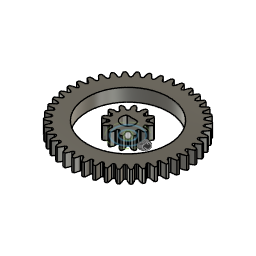
MVP miniaturisé (Autodesk Fusion 360 archive; units mm, degrees)
design "Roue dentée miniature"
description: Spur Gear; Module: 1.0; Num Teeth: 12; Pressure Angle: 20.0; Backlash: 0.00 mm
description: Spur Gear; Module: 1.0; Num Teeth: 42; Pressure Angle: 20.0; Backlash: 0.00 mm
Autodesk Fusion 360 part; units mm, degrees
(part 1 of 2)
sketch "Esquisse1" plane through (0, 0, 0) normal (0, 0, 1) x (1, 0, 0) in component "Spur Gear (12 teeth)"
  circle A0 centre (0, 0) radius 4.7492
  circle A1 centre (0, 0) radius 2.5
extrude "Extrusion1" add sketch "Esquisse1" along normal blind 4.7 makes body 1 in component "Spur Gear (12 teeth)"
sketch "Esquisse2" plane through (0, 0, 0) normal (0, 0, 1) x (1, 0, 0) in component "Spur Gear (12 teeth)"
  spline S0 degree 5 poles (5.5783, -0.8192) (5.5823, -0.8197) (5.5902, -0.8208) (5.6021, -0.8219) (5.6181, -0.8228) (5.6381, -0.8229) (5.6583, -0.8223) (5.6784, -0.8212) (5.6986, -0.8199) (5.7188, -0.8184) (5.7391, -0.8168) (5.7593, -0.8149) (5.7796, -0.8127) (5.7999, -0.8102) (5.8203, -0.8073) (5.8406, -0.8041) (5.861, -0.8006) (5.8814, -0.7969) (5.9018, -0.793) (5.9222, -0.7888) (5.9426, -0.7845) (5.9631, -0.7799) (5.9835, -0.7752) (6.0039, -0.7702) (6.0244, -0.765) (6.0448, -0.7596) (6.0653, -0.7539) (6.0857, -0.7481) (6.1061, -0.7421) (6.1266, -0.7359) (6.147, -0.7295) (6.1675, -0.7229) (6.1879, -0.7161) (6.2083, -0.7092) (6.2288, -0.7021) (6.2492, -0.6947) (6.2696, -0.6873) (6.29, -0.6796) (6.3104, -0.6717) (6.3308, -0.6637) (6.3512, -0.6555) (6.3715, -0.6472) (6.3919, -0.6387) (6.4122, -0.63) (6.4325, -0.6211) (6.4528, -0.6121) (6.4731, -0.6029) (6.4934, -0.5936) (6.5137, -0.5841) (6.5339, -0.5744) (6.5541, -0.5646) (6.5743, -0.5546) (6.5945, -0.5445) (6.6147, -0.5342) (6.6348, -0.5238) (6.655, -0.5132) (6.6751, -0.5024) (6.6951, -0.4915) (6.7152, -0.4805) (6.7352, -0.4693) (6.7552, -0.4579) (6.7752, -0.4464) (6.7952, -0.4348) (6.8151, -0.423) (6.835, -0.4111) (6.8549, -0.399) (6.8747, -0.3867) (6.8945, -0.3744) (6.9143, -0.3619) (6.9341, -0.3492) (6.9538, -0.3364) (6.9695, -0.3261) (6.9813, -0.3182) (6.9892, -0.313) (6.9931, -0.3103) knots 0 0 0 0 0 0 0.01428571 0.02857143 0.04285714 0.05714286 0.07142857 0.08571429 0.1 0.11428571 0.12857143 0.14285714 0.15714286 0.17142857 0.18571429 0.2 0.21428571 0.22857143 0.24285714 0.25714286 0.27142857 0.28571429 0.3 0.31428571 0.32857143 0.34285714 0.35714286 0.37142857 0.38571429 0.4 0.41428571 0.42857143 0.44285714 0.45714286 0.47142857 0.48571429 0.5 0.51428571 0.52857143 0.54285714 0.55714286 0.57142857 0.58571429 0.6 0.61428571 0.62857143 0.64285714 0.65714286 0.67142857 0.68571429 0.7 0.71428571 0.72857143 0.74285714 0.75714286 0.77142857 0.78571429 0.8 0.81428571 0.82857143 0.84285714 0.85714286 0.87142857 0.88571429 0.9 0.91428571 0.92857143 0.94285714 0.95714286 0.97142857 0.98571429 1 1 1 1 1 1
  spline S1 degree 5 poles (5.5783, 0.8192) (5.5823, 0.8197) (5.5902, 0.8208) (5.6021, 0.8219) (5.6181, 0.8228) (5.6381, 0.8229) (5.6583, 0.8223) (5.6784, 0.8212) (5.6986, 0.8199) (5.7188, 0.8184) (5.7391, 0.8168) (5.7593, 0.8149) (5.7796, 0.8127) (5.7999, 0.8102) (5.8203, 0.8073) (5.8406, 0.8041) (5.861, 0.8006) (5.8814, 0.7969) (5.9018, 0.793) (5.9222, 0.7888) (5.9426, 0.7845) (5.9631, 0.7799) (5.9835, 0.7752) (6.0039, 0.7702) (6.0244, 0.765) (6.0448, 0.7596) (6.0653, 0.7539) (6.0857, 0.7481) (6.1061, 0.7421) (6.1266, 0.7359) (6.147, 0.7295) (6.1675, 0.7229) (6.1879, 0.7161) (6.2083, 0.7092) (6.2288, 0.7021) (6.2492, 0.6947) (6.2696, 0.6873) (6.29, 0.6796) (6.3104, 0.6717) (6.3308, 0.6637) (6.3512, 0.6555) (6.3715, 0.6472) (6.3919, 0.6387) (6.4122, 0.63) (6.4325, 0.6211) (6.4528, 0.6121) (6.4731, 0.6029) (6.4934, 0.5936) (6.5137, 0.5841) (6.5339, 0.5744) (6.5541, 0.5646) (6.5743, 0.5546) (6.5945, 0.5445) (6.6147, 0.5342) (6.6348, 0.5238) (6.655, 0.5132) (6.6751, 0.5024) (6.6951, 0.4915) (6.7152, 0.4805) (6.7352, 0.4693) (6.7552, 0.4579) (6.7752, 0.4464) (6.7952, 0.4348) (6.8151, 0.423) (6.835, 0.4111) (6.8549, 0.399) (6.8747, 0.3867) (6.8945, 0.3744) (6.9143, 0.3619) (6.9341, 0.3492) (6.9538, 0.3364) (6.9695, 0.3261) (6.9813, 0.3182) (6.9892, 0.313) (6.9931, 0.3103) knots 0 0 0 0 0 0 0.01428571 0.02857143 0.04285714 0.05714286 0.07142857 0.08571429 0.1 0.11428571 0.12857143 0.14285714 0.15714286 0.17142857 0.18571429 0.2 0.21428571 0.22857143 0.24285714 0.25714286 0.27142857 0.28571429 0.3 0.31428571 0.32857143 0.34285714 0.35714286 0.37142857 0.38571429 0.4 0.41428571 0.42857143 0.44285714 0.45714286 0.47142857 0.48571429 0.5 0.51428571 0.52857143 0.54285714 0.55714286 0.57142857 0.58571429 0.6 0.61428571 0.62857143 0.64285714 0.65714286 0.67142857 0.68571429 0.7 0.71428571 0.72857143 0.74285714 0.75714286 0.77142857 0.78571429 0.8 0.81428571 0.82857143 0.84285714 0.85714286 0.87142857 0.88571429 0.9 0.91428571 0.92857143 0.94285714 0.95714286 0.97142857 0.98571429 1 1 1 1 1 1
  arc A0 (6.9931, -0.3103) -> (6.9931, 0.3103) centre (0, 0) ccw
  line L0 (4.6889, -0.69) -> (5.5783, -0.8192)
  line L1 (4.6889, 0.69) -> (5.5783, 0.8192)
  line L2 (4.6889, -0.69) -> (4.6889, 0.69)
  point P0 (5.6763, -0.8213)
  point P1 (5.7758, -0.8131)
  point P2 (5.8761, -0.7978)
  point P3 (5.977, -0.7767)
  point P4 (6.0784, -0.7502)
  point P5 (6.1802, -0.7187)
  point P6 (6.2821, -0.6825)
  point P7 (6.3842, -0.6419)
  point P8 (6.4862, -0.5969)
  point P9 (6.5882, -0.5477)
  point P10 (6.6899, -0.4943)
  point P11 (6.7914, -0.437)
  point P12 (6.8925, -0.3756)
  point P13 (5.6763, 0.8213)
  point P14 (5.7758, 0.8131)
  point P15 (5.8761, 0.7978)
  point P16 (5.977, 0.7767)
  point P17 (6.0784, 0.7502)
  point P18 (6.1802, 0.7187)
  point P19 (6.2821, 0.6825)
  point P20 (6.3842, 0.6419)
  point P21 (6.4862, 0.5969)
  point P22 (6.5882, 0.5477)
  point P23 (6.6899, 0.4943)
  point P24 (6.7914, 0.437)
  point P25 (6.8925, 0.3756)
extrude "Extrusion2" add sketch "Esquisse2" along normal blind 4.7 bodies 1 in component "Spur Gear (12 teeth)"
fillet "Congé1" radius 0.5 2 edges at (4.6986, -0.6914, 2.35) (4.6986, 0.6914, 2.35) on bodies 1 in component "Spur Gear (12 teeth)"
pattern_circular "Réseau C1" count 12 over 360 about axis through (0, 0, 0) along (0, 0, 1) of "Extrusion2", "Congé1" in component "Spur Gear (12 teeth)"
sketch "Esquisse3" plane through (0, 0, 0) normal (0, 0, 1) x (1, 0, 0) in component "Spur Gear (12 teeth)"
  circle A0 centre (0, 0) radius 6 construction
sketch "Esquisse2 (2)" plane through (0, 0, 0) normal (0, 0, -1) x (1, 0, 0)
  circle A0 centre (0, 0) radius 2.5
  arc A1 (3.2424, 4.0966) -> (3.2887, 3.4262) centre (3.635, 3.7869) ccw
  line L0 (3.2424, 4.0966) -> (3.4986, 4.4214)
  spline S0 degree 5 poles (3.4986, 4.4214) (3.5011, 4.4245) (3.5059, 4.4309) (3.5129, 4.4406) (3.5216, 4.454) (3.5317, 4.4713) (3.5412, 4.4891) (3.5504, 4.5071) (3.5594, 4.5252) (3.5682, 4.5434) (3.5769, 4.5618) (3.5854, 4.5803) (3.5936, 4.599) (3.6016, 4.6178) (3.6093, 4.6369) (3.6167, 4.6561) (3.6239, 4.6755) (3.6308, 4.695) (3.6376, 4.7146) (3.6442, 4.7344) (3.6507, 4.7542) (3.657, 4.7742) (3.6631, 4.7943) (3.669, 4.8144) (3.6747, 4.8348) (3.6802, 4.8552) (3.6856, 4.8757) (3.6907, 4.8963) (3.6957, 4.917) (3.7006, 4.9378) (3.7053, 4.9587) (3.7098, 4.9797) (3.7142, 5.0008) (3.7184, 5.022) (3.7224, 5.0432) (3.7263, 5.0646) (3.73, 5.086) (3.7335, 5.1075) (3.7369, 5.1291) (3.7402, 5.1508) (3.7433, 5.1725) (3.7462, 5.1943) (3.749, 5.2162) (3.7517, 5.2381) (3.7542, 5.2602) (3.7565, 5.2823) (3.7587, 5.3044) (3.7608, 5.3267) (3.7627, 5.349) (3.7644, 5.3713) (3.766, 5.3937) (3.7675, 5.4162) (3.7688, 5.4388) (3.77, 5.4614) (3.771, 5.4841) (3.7719, 5.5068) (3.7726, 5.5296) (3.7732, 5.5524) (3.7737, 5.5753) (3.774, 5.5982) (3.7742, 5.6212) (3.7742, 5.6443) (3.7741, 5.6674) (3.7739, 5.6906) (3.7735, 5.7138) (3.773, 5.737) (3.7723, 5.7603) (3.7715, 5.7836) (3.7705, 5.807) (3.7694, 5.8305) (3.7682, 5.8539) (3.7671, 5.8728) (3.7663, 5.8869) (3.7656, 5.8963) (3.7653, 5.901) knots 0 0 0 0 0 0 0.01428571 0.02857143 0.04285714 0.05714286 0.07142857 0.08571429 0.1 0.11428571 0.12857143 0.14285714 0.15714286 0.17142857 0.18571429 0.2 0.21428571 0.22857143 0.24285714 0.25714286 0.27142857 0.28571429 0.3 0.31428571 0.32857143 0.34285714 0.35714286 0.37142857 0.38571429 0.4 0.41428571 0.42857143 0.44285714 0.45714286 0.47142857 0.48571429 0.5 0.51428571 0.52857143 0.54285714 0.55714286 0.57142857 0.58571429 0.6 0.61428571 0.62857143 0.64285714 0.65714286 0.67142857 0.68571429 0.7 0.71428571 0.72857143 0.74285714 0.75714286 0.77142857 0.78571429 0.8 0.81428571 0.82857143 0.84285714 0.85714286 0.87142857 0.88571429 0.9 0.91428571 0.92857143 0.94285714 0.95714286 0.97142857 0.98571429 1 1 1 1 1 1
  arc A2 (3.7653, 5.901) -> (3.2278, 6.2114) centre (0, 0) ccw
  spline S1 degree 5 poles (2.0798, 5.2406) (2.0812, 5.2443) (2.0843, 5.2517) (2.0893, 5.2626) (2.0965, 5.2768) (2.1064, 5.2942) (2.117, 5.3113) (2.128, 5.3283) (2.1393, 5.3451) (2.1506, 5.3619) (2.1622, 5.3786) (2.174, 5.3952) (2.186, 5.4117) (2.1983, 5.428) (2.211, 5.4442) (2.2239, 5.4602) (2.2372, 5.4761) (2.2506, 5.4919) (2.2642, 5.5076) (2.278, 5.5232) (2.2919, 5.5387) (2.3061, 5.5541) (2.3204, 5.5694) (2.3349, 5.5846) (2.3497, 5.5997) (2.3646, 5.6147) (2.3797, 5.6296) (2.395, 5.6444) (2.4104, 5.6591) (2.426, 5.6737) (2.4418, 5.6882) (2.4577, 5.7026) (2.4738, 5.717) (2.49, 5.7312) (2.5064, 5.7453) (2.5229, 5.7593) (2.5396, 5.7733) (2.5565, 5.7871) (2.5735, 5.8008) (2.5906, 5.8145) (2.6079, 5.828) (2.6253, 5.8415) (2.6428, 5.8549) (2.6605, 5.8681) (2.6784, 5.8813) (2.6963, 5.8944) (2.7144, 5.9074) (2.7326, 5.9203) (2.751, 5.9331) (2.7695, 5.9458) (2.7881, 5.9584) (2.8068, 5.9709) (2.8257, 5.9833) (2.8447, 5.9956) (2.8638, 6.0078) (2.8831, 6.02) (2.9024, 6.032) (2.9219, 6.0439) (2.9415, 6.0558) (2.9612, 6.0675) (2.981, 6.0792) (3.001, 6.0907) (3.0211, 6.1022) (3.0412, 6.1135) (3.0615, 6.1248) (3.0819, 6.136) (3.1024, 6.147) (3.123, 6.158) (3.1438, 6.1689) (3.1646, 6.1797) (3.1856, 6.1903) (3.2024, 6.1988) (3.2151, 6.2051) (3.2235, 6.2093) (3.2278, 6.2114) knots 0 0 0 0 0 0 0.01428571 0.02857143 0.04285714 0.05714286 0.07142857 0.08571429 0.1 0.11428571 0.12857143 0.14285714 0.15714286 0.17142857 0.18571429 0.2 0.21428571 0.22857143 0.24285714 0.25714286 0.27142857 0.28571429 0.3 0.31428571 0.32857143 0.34285714 0.35714286 0.37142857 0.38571429 0.4 0.41428571 0.42857143 0.44285714 0.45714286 0.47142857 0.48571429 0.5 0.51428571 0.52857143 0.54285714 0.55714286 0.57142857 0.58571429 0.6 0.61428571 0.62857143 0.64285714 0.65714286 0.67142857 0.68571429 0.7 0.71428571 0.72857143 0.74285714 0.75714286 0.77142857 0.78571429 0.8 0.81428571 0.82857143 0.84285714 0.85714286 0.87142857 0.88571429 0.9 0.91428571 0.92857143 0.94285714 0.95714286 0.97142857 0.98571429 1 1 1 1 1 1
  line L1 (2.0798, 5.2406) -> (1.9265, 4.8563)
  arc A3 (1.3228, 4.5613) -> (1.9265, 4.8563) centre (1.4621, 5.0415) ccw
  arc A4 (1.3228, 4.5613) -> (1.135, 4.6116) centre (0, 0) ccw
  arc A5 (0.7597, 5.1689) -> (1.135, 4.6116) centre (1.2545, 5.0971) ccw
  line L2 (0.7597, 5.1689) -> (0.8192, 5.5783)
  spline S2 degree 5 poles (0.8192, 5.5783) (0.8197, 5.5823) (0.8208, 5.5902) (0.8219, 5.6021) (0.8228, 5.6181) (0.8229, 5.6381) (0.8223, 5.6583) (0.8212, 5.6784) (0.8199, 5.6986) (0.8184, 5.7188) (0.8168, 5.7391) (0.8149, 5.7593) (0.8127, 5.7796) (0.8102, 5.7999) (0.8073, 5.8203) (0.8041, 5.8406) (0.8006, 5.861) (0.7969, 5.8814) (0.793, 5.9018) (0.7888, 5.9222) (0.7845, 5.9426) (0.7799, 5.9631) (0.7752, 5.9835) (0.7702, 6.0039) (0.765, 6.0244) (0.7596, 6.0448) (0.7539, 6.0653) (0.7481, 6.0857) (0.7421, 6.1061) (0.7359, 6.1266) (0.7295, 6.147) (0.7229, 6.1675) (0.7161, 6.1879) (0.7092, 6.2083) (0.7021, 6.2288) (0.6947, 6.2492) (0.6873, 6.2696) (0.6796, 6.29) (0.6717, 6.3104) (0.6637, 6.3308) (0.6555, 6.3512) (0.6472, 6.3715) (0.6387, 6.3919) (0.63, 6.4122) (0.6211, 6.4325) (0.6121, 6.4528) (0.6029, 6.4731) (0.5936, 6.4934) (0.5841, 6.5137) (0.5744, 6.5339) (0.5646, 6.5541) (0.5546, 6.5743) (0.5445, 6.5945) (0.5342, 6.6147) (0.5238, 6.6348) (0.5132, 6.655) (0.5024, 6.6751) (0.4915, 6.6951) (0.4805, 6.7152) (0.4693, 6.7352) (0.4579, 6.7552) (0.4464, 6.7752) (0.4348, 6.7952) (0.423, 6.8151) (0.4111, 6.835) (0.399, 6.8549) (0.3867, 6.8747) (0.3744, 6.8945) (0.3619, 6.9143) (0.3492, 6.9341) (0.3364, 6.9538) (0.3261, 6.9695) (0.3182, 6.9813) (0.313, 6.9892) (0.3103, 6.9931) knots 0 0 0 0 0 0 0.01428571 0.02857143 0.04285714 0.05714286 0.07142857 0.08571429 0.1 0.11428571 0.12857143 0.14285714 0.15714286 0.17142857 0.18571429 0.2 0.21428571 0.22857143 0.24285714 0.25714286 0.27142857 0.28571429 0.3 0.31428571 0.32857143 0.34285714 0.35714286 0.37142857 0.38571429 0.4 0.41428571 0.42857143 0.44285714 0.45714286 0.47142857 0.48571429 0.5 0.51428571 0.52857143 0.54285714 0.55714286 0.57142857 0.58571429 0.6 0.61428571 0.62857143 0.64285714 0.65714286 0.67142857 0.68571429 0.7 0.71428571 0.72857143 0.74285714 0.75714286 0.77142857 0.78571429 0.8 0.81428571 0.82857143 0.84285714 0.85714286 0.87142857 0.88571429 0.9 0.91428571 0.92857143 0.94285714 0.95714286 0.97142857 0.98571429 1 1 1 1 1 1
  arc A6 (0.3103, 6.9931) -> (-0.3103, 6.9931) centre (0, 0) ccw
  spline S3 degree 5 poles (-0.8192, 5.5783) (-0.8197, 5.5823) (-0.8208, 5.5902) (-0.8219, 5.6021) (-0.8228, 5.6181) (-0.8229, 5.6381) (-0.8223, 5.6583) (-0.8212, 5.6784) (-0.8199, 5.6986) (-0.8184, 5.7188) (-0.8168, 5.7391) (-0.8149, 5.7593) (-0.8127, 5.7796) (-0.8102, 5.7999) (-0.8073, 5.8203) (-0.8041, 5.8406) (-0.8006, 5.861) (-0.7969, 5.8814) (-0.793, 5.9018) (-0.7888, 5.9222) (-0.7845, 5.9426) (-0.7799, 5.9631) (-0.7752, 5.9835) (-0.7702, 6.0039) (-0.765, 6.0244) (-0.7596, 6.0448) (-0.7539, 6.0653) (-0.7481, 6.0857) (-0.7421, 6.1061) (-0.7359, 6.1266) (-0.7295, 6.147) (-0.7229, 6.1675) (-0.7161, 6.1879) (-0.7092, 6.2083) (-0.7021, 6.2288) (-0.6947, 6.2492) (-0.6873, 6.2696) (-0.6796, 6.29) (-0.6717, 6.3104) (-0.6637, 6.3308) (-0.6555, 6.3512) (-0.6472, 6.3715) (-0.6387, 6.3919) (-0.63, 6.4122) (-0.6211, 6.4325) (-0.6121, 6.4528) (-0.6029, 6.4731) (-0.5936, 6.4934) (-0.5841, 6.5137) (-0.5744, 6.5339) (-0.5646, 6.5541) (-0.5546, 6.5743) (-0.5445, 6.5945) (-0.5342, 6.6147) (-0.5238, 6.6348) (-0.5132, 6.655) (-0.5024, 6.6751) (-0.4915, 6.6951) (-0.4805, 6.7152) (-0.4693, 6.7352) (-0.4579, 6.7552) (-0.4464, 6.7752) (-0.4348, 6.7952) (-0.423, 6.8151) (-0.4111, 6.835) (-0.399, 6.8549) (-0.3867, 6.8747) (-0.3744, 6.8945) (-0.3619, 6.9143) (-0.3492, 6.9341) (-0.3364, 6.9538) (-0.3261, 6.9695) (-0.3182, 6.9813) (-0.313, 6.9892) (-0.3103, 6.9931) knots 0 0 0 0 0 0 0.01428571 0.02857143 0.04285714 0.05714286 0.07142857 0.08571429 0.1 0.11428571 0.12857143 0.14285714 0.15714286 0.17142857 0.18571429 0.2 0.21428571 0.22857143 0.24285714 0.25714286 0.27142857 0.28571429 0.3 0.31428571 0.32857143 0.34285714 0.35714286 0.37142857 0.38571429 0.4 0.41428571 0.42857143 0.44285714 0.45714286 0.47142857 0.48571429 0.5 0.51428571 0.52857143 0.54285714 0.55714286 0.57142857 0.58571429 0.6 0.61428571 0.62857143 0.64285714 0.65714286 0.67142857 0.68571429 0.7 0.71428571 0.72857143 0.74285714 0.75714286 0.77142857 0.78571429 0.8 0.81428571 0.82857143 0.84285714 0.85714286 0.87142857 0.88571429 0.9 0.91428571 0.92857143 0.94285714 0.95714286 0.97142857 0.98571429 1 1 1 1 1 1
  line L3 (-0.8192, 5.5783) -> (-0.7597, 5.1689)
  arc A7 (-1.135, 4.6116) -> (-0.7597, 5.1689) centre (-1.2545, 5.0971) ccw
  arc A8 (-1.135, 4.6116) -> (-1.3228, 4.5613) centre (0, 0) ccw
  arc A9 (-1.9265, 4.8563) -> (-1.3228, 4.5613) centre (-1.4621, 5.0415) ccw
  line L4 (-1.9265, 4.8563) -> (-2.0798, 5.2406)
  spline S4 degree 5 poles (-2.0798, 5.2406) (-2.0812, 5.2443) (-2.0843, 5.2517) (-2.0893, 5.2626) (-2.0965, 5.2768) (-2.1064, 5.2942) (-2.117, 5.3113) (-2.128, 5.3283) (-2.1393, 5.3451) (-2.1506, 5.3619) (-2.1622, 5.3786) (-2.174, 5.3952) (-2.186, 5.4117) (-2.1983, 5.428) (-2.211, 5.4442) (-2.2239, 5.4602) (-2.2372, 5.4761) (-2.2506, 5.4919) (-2.2642, 5.5076) (-2.278, 5.5232) (-2.2919, 5.5387) (-2.3061, 5.5541) (-2.3204, 5.5694) (-2.3349, 5.5846) (-2.3497, 5.5997) (-2.3646, 5.6147) (-2.3797, 5.6296) (-2.395, 5.6444) (-2.4104, 5.6591) (-2.426, 5.6737) (-2.4418, 5.6882) (-2.4577, 5.7026) (-2.4738, 5.717) (-2.49, 5.7312) (-2.5064, 5.7453) (-2.5229, 5.7593) (-2.5396, 5.7733) (-2.5565, 5.7871) (-2.5735, 5.8008) (-2.5906, 5.8145) (-2.6079, 5.828) (-2.6253, 5.8415) (-2.6428, 5.8549) (-2.6605, 5.8681) (-2.6784, 5.8813) (-2.6963, 5.8944) (-2.7144, 5.9074) (-2.7326, 5.9203) (-2.751, 5.9331) (-2.7695, 5.9458) (-2.7881, 5.9584) (-2.8068, 5.9709) (-2.8257, 5.9833) (-2.8447, 5.9956) (-2.8638, 6.0078) (-2.8831, 6.02) (-2.9024, 6.032) (-2.9219, 6.0439) (-2.9415, 6.0558) (-2.9612, 6.0675) (-2.981, 6.0792) (-3.001, 6.0907) (-3.0211, 6.1022) (-3.0412, 6.1135) (-3.0615, 6.1248) (-3.0819, 6.136) (-3.1024, 6.147) (-3.123, 6.158) (-3.1438, 6.1689) (-3.1646, 6.1797) (-3.1856, 6.1903) (-3.2024, 6.1988) (-3.2151, 6.2051) (-3.2235, 6.2093) (-3.2278, 6.2114) knots 0 0 0 0 0 0 0.01428571 0.02857143 0.04285714 0.05714286 0.07142857 0.08571429 0.1 0.11428571 0.12857143 0.14285714 0.15714286 0.17142857 0.18571429 0.2 0.21428571 0.22857143 0.24285714 0.25714286 0.27142857 0.28571429 0.3 0.31428571 0.32857143 0.34285714 0.35714286 0.37142857 0.38571429 0.4 0.41428571 0.42857143 0.44285714 0.45714286 0.47142857 0.48571429 0.5 0.51428571 0.52857143 0.54285714 0.55714286 0.57142857 0.58571429 0.6 0.61428571 0.62857143 0.64285714 0.65714286 0.67142857 0.68571429 0.7 0.71428571 0.72857143 0.74285714 0.75714286 0.77142857 0.78571429 0.8 0.81428571 0.82857143 0.84285714 0.85714286 0.87142857 0.88571429 0.9 0.91428571 0.92857143 0.94285714 0.95714286 0.97142857 0.98571429 1 1 1 1 1 1
  arc A10 (-3.2278, 6.2114) -> (-3.7653, 5.901) centre (0, 0) ccw
  spline S5 degree 5 poles (-3.4986, 4.4214) (-3.5011, 4.4245) (-3.5059, 4.4309) (-3.5129, 4.4406) (-3.5216, 4.454) (-3.5317, 4.4713) (-3.5412, 4.4891) (-3.5504, 4.5071) (-3.5594, 4.5252) (-3.5682, 4.5434) (-3.5769, 4.5618) (-3.5854, 4.5803) (-3.5936, 4.599) (-3.6016, 4.6178) (-3.6093, 4.6369) (-3.6167, 4.6561) (-3.6239, 4.6755) (-3.6308, 4.695) (-3.6376, 4.7146) (-3.6442, 4.7344) (-3.6507, 4.7542) (-3.657, 4.7742) (-3.6631, 4.7943) (-3.669, 4.8144) (-3.6747, 4.8348) (-3.6802, 4.8552) (-3.6856, 4.8757) (-3.6907, 4.8963) (-3.6957, 4.917) (-3.7006, 4.9378) (-3.7053, 4.9587) (-3.7098, 4.9797) (-3.7142, 5.0008) (-3.7184, 5.022) (-3.7224, 5.0432) (-3.7263, 5.0646) (-3.73, 5.086) (-3.7335, 5.1075) (-3.7369, 5.1291) (-3.7402, 5.1508) (-3.7433, 5.1725) (-3.7462, 5.1943) (-3.749, 5.2162) (-3.7517, 5.2381) (-3.7542, 5.2602) (-3.7565, 5.2823) (-3.7587, 5.3044) (-3.7608, 5.3267) (-3.7627, 5.349) (-3.7644, 5.3713) (-3.766, 5.3937) (-3.7675, 5.4162) (-3.7688, 5.4388) (-3.77, 5.4614) (-3.771, 5.4841) (-3.7719, 5.5068) (-3.7726, 5.5296) (-3.7732, 5.5524) (-3.7737, 5.5753) (-3.774, 5.5982) (-3.7742, 5.6212) (-3.7742, 5.6443) (-3.7741, 5.6674) (-3.7739, 5.6906) (-3.7735, 5.7138) (-3.773, 5.737) (-3.7723, 5.7603) (-3.7715, 5.7836) (-3.7705, 5.807) (-3.7694, 5.8305) (-3.7682, 5.8539) (-3.7671, 5.8728) (-3.7663, 5.8869) (-3.7656, 5.8963) (-3.7653, 5.901) knots 0 0 0 0 0 0 0.01428571 0.02857143 0.04285714 0.05714286 0.07142857 0.08571429 0.1 0.11428571 0.12857143 0.14285714 0.15714286 0.17142857 0.18571429 0.2 0.21428571 0.22857143 0.24285714 0.25714286 0.27142857 0.28571429 0.3 0.31428571 0.32857143 0.34285714 0.35714286 0.37142857 0.38571429 0.4 0.41428571 0.42857143 0.44285714 0.45714286 0.47142857 0.48571429 0.5 0.51428571 0.52857143 0.54285714 0.55714286 0.57142857 0.58571429 0.6 0.61428571 0.62857143 0.64285714 0.65714286 0.67142857 0.68571429 0.7 0.71428571 0.72857143 0.74285714 0.75714286 0.77142857 0.78571429 0.8 0.81428571 0.82857143 0.84285714 0.85714286 0.87142857 0.88571429 0.9 0.91428571 0.92857143 0.94285714 0.95714286 0.97142857 0.98571429 1 1 1 1 1 1
  line L5 (-3.4986, 4.4214) -> (-3.2424, 4.0966)
  arc A11 (-3.2887, 3.4262) -> (-3.2424, 4.0966) centre (-3.635, 3.7869) ccw
  arc A12 (-3.2887, 3.4262) -> (-3.4262, 3.2887) centre (0, 0) ccw
  arc A13 (-4.0966, 3.2424) -> (-3.4262, 3.2887) centre (-3.7869, 3.635) ccw
  line L6 (-4.0966, 3.2424) -> (-4.4214, 3.4986)
  spline S6 degree 5 poles (-4.4214, 3.4986) (-4.4245, 3.5011) (-4.4309, 3.5059) (-4.4406, 3.5129) (-4.454, 3.5216) (-4.4713, 3.5317) (-4.4891, 3.5412) (-4.5071, 3.5504) (-4.5252, 3.5594) (-4.5434, 3.5682) (-4.5618, 3.5769) (-4.5803, 3.5854) (-4.599, 3.5936) (-4.6178, 3.6016) (-4.6369, 3.6093) (-4.6561, 3.6167) (-4.6755, 3.6239) (-4.695, 3.6308) (-4.7146, 3.6376) (-4.7344, 3.6442) (-4.7542, 3.6507) (-4.7742, 3.657) (-4.7943, 3.6631) (-4.8144, 3.669) (-4.8348, 3.6747) (-4.8552, 3.6802) (-4.8757, 3.6856) (-4.8963, 3.6907) (-4.917, 3.6957) (-4.9378, 3.7006) (-4.9587, 3.7053) (-4.9797, 3.7098) (-5.0008, 3.7142) (-5.022, 3.7184) (-5.0432, 3.7224) (-5.0646, 3.7263) (-5.086, 3.73) (-5.1075, 3.7335) (-5.1291, 3.7369) (-5.1508, 3.7402) (-5.1725, 3.7433) (-5.1943, 3.7462) (-5.2162, 3.749) (-5.2381, 3.7517) (-5.2602, 3.7542) (-5.2823, 3.7565) (-5.3044, 3.7587) (-5.3267, 3.7608) (-5.349, 3.7627) (-5.3713, 3.7644) (-5.3937, 3.766) (-5.4162, 3.7675) (-5.4388, 3.7688) (-5.4614, 3.77) (-5.4841, 3.771) (-5.5068, 3.7719) (-5.5296, 3.7726) (-5.5524, 3.7732) (-5.5753, 3.7737) (-5.5982, 3.774) (-5.6212, 3.7742) (-5.6443, 3.7742) (-5.6674, 3.7741) (-5.6906, 3.7739) (-5.7138, 3.7735) (-5.737, 3.773) (-5.7603, 3.7723) (-5.7836, 3.7715) (-5.807, 3.7705) (-5.8305, 3.7694) (-5.8539, 3.7682) (-5.8728, 3.7671) (-5.8869, 3.7663) (-5.8963, 3.7656) (-5.901, 3.7653) knots 0 0 0 0 0 0 0.01428571 0.02857143 0.04285714 0.05714286 0.07142857 0.08571429 0.1 0.11428571 0.12857143 0.14285714 0.15714286 0.17142857 0.18571429 0.2 0.21428571 0.22857143 0.24285714 0.25714286 0.27142857 0.28571429 0.3 0.31428571 0.32857143 0.34285714 0.35714286 0.37142857 0.38571429 0.4 0.41428571 0.42857143 0.44285714 0.45714286 0.47142857 0.48571429 0.5 0.51428571 0.52857143 0.54285714 0.55714286 0.57142857 0.58571429 0.6 0.61428571 0.62857143 0.64285714 0.65714286 0.67142857 0.68571429 0.7 0.71428571 0.72857143 0.74285714 0.75714286 0.77142857 0.78571429 0.8 0.81428571 0.82857143 0.84285714 0.85714286 0.87142857 0.88571429 0.9 0.91428571 0.92857143 0.94285714 0.95714286 0.97142857 0.98571429 1 1 1 1 1 1
  arc A14 (-5.901, 3.7653) -> (-6.2114, 3.2278) centre (0, 0) ccw
  spline S7 degree 5 poles (-5.2406, 2.0798) (-5.2443, 2.0812) (-5.2517, 2.0843) (-5.2626, 2.0893) (-5.2768, 2.0965) (-5.2942, 2.1064) (-5.3113, 2.117) (-5.3283, 2.128) (-5.3451, 2.1393) (-5.3619, 2.1506) (-5.3786, 2.1622) (-5.3952, 2.174) (-5.4117, 2.186) (-5.428, 2.1983) (-5.4442, 2.211) (-5.4602, 2.2239) (-5.4761, 2.2372) (-5.4919, 2.2506) (-5.5076, 2.2642) (-5.5232, 2.278) (-5.5387, 2.2919) (-5.5541, 2.3061) (-5.5694, 2.3204) (-5.5846, 2.3349) (-5.5997, 2.3497) (-5.6147, 2.3646) (-5.6296, 2.3797) (-5.6444, 2.395) (-5.6591, 2.4104) (-5.6737, 2.426) (-5.6882, 2.4418) (-5.7026, 2.4577) (-5.717, 2.4738) (-5.7312, 2.49) (-5.7453, 2.5064) (-5.7593, 2.5229) (-5.7733, 2.5396) (-5.7871, 2.5565) (-5.8008, 2.5735) (-5.8145, 2.5906) (-5.828, 2.6079) (-5.8415, 2.6253) (-5.8549, 2.6428) (-5.8681, 2.6605) (-5.8813, 2.6784) (-5.8944, 2.6963) (-5.9074, 2.7144) (-5.9203, 2.7326) (-5.9331, 2.751) (-5.9458, 2.7695) (-5.9584, 2.7881) (-5.9709, 2.8068) (-5.9833, 2.8257) (-5.9956, 2.8447) (-6.0078, 2.8638) (-6.02, 2.8831) (-6.032, 2.9024) (-6.0439, 2.9219) (-6.0558, 2.9415) (-6.0675, 2.9612) (-6.0792, 2.981) (-6.0907, 3.001) (-6.1022, 3.0211) (-6.1135, 3.0412) (-6.1248, 3.0615) (-6.136, 3.0819) (-6.147, 3.1024) (-6.158, 3.123) (-6.1689, 3.1438) (-6.1797, 3.1646) (-6.1903, 3.1856) (-6.1988, 3.2024) (-6.2051, 3.2151) (-6.2093, 3.2235) (-6.2114, 3.2278) knots 0 0 0 0 0 0 0.01428571 0.02857143 0.04285714 0.05714286 0.07142857 0.08571429 0.1 0.11428571 0.12857143 0.14285714 0.15714286 0.17142857 0.18571429 0.2 0.21428571 0.22857143 0.24285714 0.25714286 0.27142857 0.28571429 0.3 0.31428571 0.32857143 0.34285714 0.35714286 0.37142857 0.38571429 0.4 0.41428571 0.42857143 0.44285714 0.45714286 0.47142857 0.48571429 0.5 0.51428571 0.52857143 0.54285714 0.55714286 0.57142857 0.58571429 0.6 0.61428571 0.62857143 0.64285714 0.65714286 0.67142857 0.68571429 0.7 0.71428571 0.72857143 0.74285714 0.75714286 0.77142857 0.78571429 0.8 0.81428571 0.82857143 0.84285714 0.85714286 0.87142857 0.88571429 0.9 0.91428571 0.92857143 0.94285714 0.95714286 0.97142857 0.98571429 1 1 1 1 1 1
  line L7 (-5.2406, 2.0798) -> (-4.8563, 1.9265)
  arc A15 (-4.5613, 1.3228) -> (-4.8563, 1.9265) centre (-5.0415, 1.4621) ccw
  arc A16 (-4.5613, 1.3228) -> (-4.6116, 1.135) centre (0, 0) ccw
  arc A17 (-5.1689, 0.7597) -> (-4.6116, 1.135) centre (-5.0971, 1.2545) ccw
  line L8 (-5.1689, 0.7597) -> (-5.5783, 0.8192)
  spline S8 degree 5 poles (-5.5783, 0.8192) (-5.5823, 0.8197) (-5.5902, 0.8208) (-5.6021, 0.8219) (-5.6181, 0.8228) (-5.6381, 0.8229) (-5.6583, 0.8223) (-5.6784, 0.8212) (-5.6986, 0.8199) (-5.7188, 0.8184) (-5.7391, 0.8168) (-5.7593, 0.8149) (-5.7796, 0.8127) (-5.7999, 0.8102) (-5.8203, 0.8073) (-5.8406, 0.8041) (-5.861, 0.8006) (-5.8814, 0.7969) (-5.9018, 0.793) (-5.9222, 0.7888) (-5.9426, 0.7845) (-5.9631, 0.7799) (-5.9835, 0.7752) (-6.0039, 0.7702) (-6.0244, 0.765) (-6.0448, 0.7596) (-6.0653, 0.7539) (-6.0857, 0.7481) (-6.1061, 0.7421) (-6.1266, 0.7359) (-6.147, 0.7295) (-6.1675, 0.7229) (-6.1879, 0.7161) (-6.2083, 0.7092) (-6.2288, 0.7021) (-6.2492, 0.6947) (-6.2696, 0.6873) (-6.29, 0.6796) (-6.3104, 0.6717) (-6.3308, 0.6637) (-6.3512, 0.6555) (-6.3715, 0.6472) (-6.3919, 0.6387) (-6.4122, 0.63) (-6.4325, 0.6211) (-6.4528, 0.6121) (-6.4731, 0.6029) (-6.4934, 0.5936) (-6.5137, 0.5841) (-6.5339, 0.5744) (-6.5541, 0.5646) (-6.5743, 0.5546) (-6.5945, 0.5445) (-6.6147, 0.5342) (-6.6348, 0.5238) (-6.655, 0.5132) (-6.6751, 0.5024) (-6.6951, 0.4915) (-6.7152, 0.4805) (-6.7352, 0.4693) (-6.7552, 0.4579) (-6.7752, 0.4464) (-6.7952, 0.4348) (-6.8151, 0.423) (-6.835, 0.4111) (-6.8549, 0.399) (-6.8747, 0.3867) (-6.8945, 0.3744) (-6.9143, 0.3619) (-6.9341, 0.3492) (-6.9538, 0.3364) (-6.9695, 0.3261) (-6.9813, 0.3182) (-6.9892, 0.313) (-6.9931, 0.3103) knots 0 0 0 0 0 0 0.01428571 0.02857143 0.04285714 0.05714286 0.07142857 0.08571429 0.1 0.11428571 0.12857143 0.14285714 0.15714286 0.17142857 0.18571429 0.2 0.21428571 0.22857143 0.24285714 0.25714286 0.27142857 0.28571429 0.3 0.31428571 0.32857143 0.34285714 0.35714286 0.37142857 0.38571429 0.4 0.41428571 0.42857143 0.44285714 0.45714286 0.47142857 0.48571429 0.5 0.51428571 0.52857143 0.54285714 0.55714286 0.57142857 0.58571429 0.6 0.61428571 0.62857143 0.64285714 0.65714286 0.67142857 0.68571429 0.7 0.71428571 0.72857143 0.74285714 0.75714286 0.77142857 0.78571429 0.8 0.81428571 0.82857143 0.84285714 0.85714286 0.87142857 0.88571429 0.9 0.91428571 0.92857143 0.94285714 0.95714286 0.97142857 0.98571429 1 1 1 1 1 1
  arc A18 (-6.9931, 0.3103) -> (-6.9931, -0.3103) centre (0, 0) ccw
  spline S9 degree 5 poles (-5.5783, -0.8192) (-5.5823, -0.8197) (-5.5902, -0.8208) (-5.6021, -0.8219) (-5.6181, -0.8228) (-5.6381, -0.8229) (-5.6583, -0.8223) (-5.6784, -0.8212) (-5.6986, -0.8199) (-5.7188, -0.8184) (-5.7391, -0.8168) (-5.7593, -0.8149) (-5.7796, -0.8127) (-5.7999, -0.8102) (-5.8203, -0.8073) (-5.8406, -0.8041) (-5.861, -0.8006) (-5.8814, -0.7969) (-5.9018, -0.793) (-5.9222, -0.7888) (-5.9426, -0.7845) (-5.9631, -0.7799) (-5.9835, -0.7752) (-6.0039, -0.7702) (-6.0244, -0.765) (-6.0448, -0.7596) (-6.0653, -0.7539) (-6.0857, -0.7481) (-6.1061, -0.7421) (-6.1266, -0.7359) (-6.147, -0.7295) (-6.1675, -0.7229) (-6.1879, -0.7161) (-6.2083, -0.7092) (-6.2288, -0.7021) (-6.2492, -0.6947) (-6.2696, -0.6873) (-6.29, -0.6796) (-6.3104, -0.6717) (-6.3308, -0.6637) (-6.3512, -0.6555) (-6.3715, -0.6472) (-6.3919, -0.6387) (-6.4122, -0.63) (-6.4325, -0.6211) (-6.4528, -0.6121) (-6.4731, -0.6029) (-6.4934, -0.5936) (-6.5137, -0.5841) (-6.5339, -0.5744) (-6.5541, -0.5646) (-6.5743, -0.5546) (-6.5945, -0.5445) (-6.6147, -0.5342) (-6.6348, -0.5238) (-6.655, -0.5132) (-6.6751, -0.5024) (-6.6951, -0.4915) (-6.7152, -0.4805) (-6.7352, -0.4693) (-6.7552, -0.4579) (-6.7752, -0.4464) (-6.7952, -0.4348) (-6.8151, -0.423) (-6.835, -0.4111) (-6.8549, -0.399) (-6.8747, -0.3867) (-6.8945, -0.3744) (-6.9143, -0.3619) (-6.9341, -0.3492) (-6.9538, -0.3364) (-6.9695, -0.3261) (-6.9813, -0.3182) (-6.9892, -0.313) (-6.9931, -0.3103) knots 0 0 0 0 0 0 0.01428571 0.02857143 0.04285714 0.05714286 0.07142857 0.08571429 0.1 0.11428571 0.12857143 0.14285714 0.15714286 0.17142857 0.18571429 0.2 0.21428571 0.22857143 0.24285714 0.25714286 0.27142857 0.28571429 0.3 0.31428571 0.32857143 0.34285714 0.35714286 0.37142857 0.38571429 0.4 0.41428571 0.42857143 0.44285714 0.45714286 0.47142857 0.48571429 0.5 0.51428571 0.52857143 0.54285714 0.55714286 0.57142857 0.58571429 0.6 0.61428571 0.62857143 0.64285714 0.65714286 0.67142857 0.68571429 0.7 0.71428571 0.72857143 0.74285714 0.75714286 0.77142857 0.78571429 0.8 0.81428571 0.82857143 0.84285714 0.85714286 0.87142857 0.88571429 0.9 0.91428571 0.92857143 0.94285714 0.95714286 0.97142857 0.98571429 1 1 1 1 1 1
  line L9 (-5.5783, -0.8192) -> (-5.1689, -0.7597)
  arc A19 (-4.6116, -1.135) -> (-5.1689, -0.7597) centre (-5.0971, -1.2545) ccw
  arc A20 (-4.6116, -1.135) -> (-4.5613, -1.3228) centre (0, 0) ccw
  arc A21 (-4.8563, -1.9265) -> (-4.5613, -1.3228) centre (-5.0415, -1.4621) ccw
  line L10 (-4.8563, -1.9265) -> (-5.2406, -2.0798)
  spline S10 degree 5 poles (-5.2406, -2.0798) (-5.2443, -2.0812) (-5.2517, -2.0843) (-5.2626, -2.0893) (-5.2768, -2.0965) (-5.2942, -2.1064) (-5.3113, -2.117) (-5.3283, -2.128) (-5.3451, -2.1393) (-5.3619, -2.1506) (-5.3786, -2.1622) (-5.3952, -2.174) (-5.4117, -2.186) (-5.428, -2.1983) (-5.4442, -2.211) (-5.4602, -2.2239) (-5.4761, -2.2372) (-5.4919, -2.2506) (-5.5076, -2.2642) (-5.5232, -2.278) (-5.5387, -2.2919) (-5.5541, -2.3061) (-5.5694, -2.3204) (-5.5846, -2.3349) (-5.5997, -2.3497) (-5.6147, -2.3646) (-5.6296, -2.3797) (-5.6444, -2.395) (-5.6591, -2.4104) (-5.6737, -2.426) (-5.6882, -2.4418) (-5.7026, -2.4577) (-5.717, -2.4738) (-5.7312, -2.49) (-5.7453, -2.5064) (-5.7593, -2.5229) (-5.7733, -2.5396) (-5.7871, -2.5565) (-5.8008, -2.5735) (-5.8145, -2.5906) (-5.828, -2.6079) (-5.8415, -2.6253) (-5.8549, -2.6428) (-5.8681, -2.6605) (-5.8813, -2.6784) (-5.8944, -2.6963) (-5.9074, -2.7144) (-5.9203, -2.7326) (-5.9331, -2.751) (-5.9458, -2.7695) (-5.9584, -2.7881) (-5.9709, -2.8068) (-5.9833, -2.8257) (-5.9956, -2.8447) (-6.0078, -2.8638) (-6.02, -2.8831) (-6.032, -2.9024) (-6.0439, -2.9219) (-6.0558, -2.9415) (-6.0675, -2.9612) (-6.0792, -2.981) (-6.0907, -3.001) (-6.1022, -3.0211) (-6.1135, -3.0412) (-6.1248, -3.0615) (-6.136, -3.0819) (-6.147, -3.1024) (-6.158, -3.123) (-6.1689, -3.1438) (-6.1797, -3.1646) (-6.1903, -3.1856) (-6.1988, -3.2024) (-6.2051, -3.2151) (-6.2093, -3.2235) (-6.2114, -3.2278) knots 0 0 0 0 0 0 0.01428571 0.02857143 0.04285714 0.05714286 0.07142857 0.08571429 0.1 0.11428571 0.12857143 0.14285714 0.15714286 0.17142857 0.18571429 0.2 0.21428571 0.22857143 0.24285714 0.25714286 0.27142857 0.28571429 0.3 0.31428571 0.32857143 0.34285714 0.35714286 0.37142857 0.38571429 0.4 0.41428571 0.42857143 0.44285714 0.45714286 0.47142857 0.48571429 0.5 0.51428571 0.52857143 0.54285714 0.55714286 0.57142857 0.58571429 0.6 0.61428571 0.62857143 0.64285714 0.65714286 0.67142857 0.68571429 0.7 0.71428571 0.72857143 0.74285714 0.75714286 0.77142857 0.78571429 0.8 0.81428571 0.82857143 0.84285714 0.85714286 0.87142857 0.88571429 0.9 0.91428571 0.92857143 0.94285714 0.95714286 0.97142857 0.98571429 1 1 1 1 1 1
  arc A22 (-6.2114, -3.2278) -> (-5.901, -3.7653) centre (0, 0) ccw
  spline S11 degree 5 poles (-4.4214, -3.4986) (-4.4245, -3.5011) (-4.4309, -3.5059) (-4.4406, -3.5129) (-4.454, -3.5216) (-4.4713, -3.5317) (-4.4891, -3.5412) (-4.5071, -3.5504) (-4.5252, -3.5594) (-4.5434, -3.5682) (-4.5618, -3.5769) (-4.5803, -3.5854) (-4.599, -3.5936) (-4.6178, -3.6016) (-4.6369, -3.6093) (-4.6561, -3.6167) (-4.6755, -3.6239) (-4.695, -3.6308) (-4.7146, -3.6376) (-4.7344, -3.6442) (-4.7542, -3.6507) (-4.7742, -3.657) (-4.7943, -3.6631) (-4.8144, -3.669) (-4.8348, -3.6747) (-4.8552, -3.6802) (-4.8757, -3.6856) (-4.8963, -3.6907) (-4.917, -3.6957) (-4.9378, -3.7006) (-4.9587, -3.7053) (-4.9797, -3.7098) (-5.0008, -3.7142) (-5.022, -3.7184) (-5.0432, -3.7224) (-5.0646, -3.7263) (-5.086, -3.73) (-5.1075, -3.7335) (-5.1291, -3.7369) (-5.1508, -3.7402) (-5.1725, -3.7433) (-5.1943, -3.7462) (-5.2162, -3.749) (-5.2381, -3.7517) (-5.2602, -3.7542) (-5.2823, -3.7565) (-5.3044, -3.7587) (-5.3267, -3.7608) (-5.349, -3.7627) (-5.3713, -3.7644) (-5.3937, -3.766) (-5.4162, -3.7675) (-5.4388, -3.7688) (-5.4614, -3.77) (-5.4841, -3.771) (-5.5068, -3.7719) (-5.5296, -3.7726) (-5.5524, -3.7732) (-5.5753, -3.7737) (-5.5982, -3.774) (-5.6212, -3.7742) (-5.6443, -3.7742) (-5.6674, -3.7741) (-5.6906, -3.7739) (-5.7138, -3.7735) (-5.737, -3.773) (-5.7603, -3.7723) (-5.7836, -3.7715) (-5.807, -3.7705) (-5.8305, -3.7694) (-5.8539, -3.7682) (-5.8728, -3.7671) (-5.8869, -3.7663) (-5.8963, -3.7656) (-5.901, -3.7653) knots 0 0 0 0 0 0 0.01428571 0.02857143 0.04285714 0.05714286 0.07142857 0.08571429 0.1 0.11428571 0.12857143 0.14285714 0.15714286 0.17142857 0.18571429 0.2 0.21428571 0.22857143 0.24285714 0.25714286 0.27142857 0.28571429 0.3 0.31428571 0.32857143 0.34285714 0.35714286 0.37142857 0.38571429 0.4 0.41428571 0.42857143 0.44285714 0.45714286 0.47142857 0.48571429 0.5 0.51428571 0.52857143 0.54285714 0.55714286 0.57142857 0.58571429 0.6 0.61428571 0.62857143 0.64285714 0.65714286 0.67142857 0.68571429 0.7 0.71428571 0.72857143 0.74285714 0.75714286 0.77142857 0.78571429 0.8 0.81428571 0.82857143 0.84285714 0.85714286 0.87142857 0.88571429 0.9 0.91428571 0.92857143 0.94285714 0.95714286 0.97142857 0.98571429 1 1 1 1 1 1
  line L11 (-4.4214, -3.4986) -> (-4.0966, -3.2424)
  arc A23 (-3.4262, -3.2887) -> (-4.0966, -3.2424) centre (-3.7869, -3.635) ccw
  arc A24 (-3.4262, -3.2887) -> (-3.2887, -3.4262) centre (0, 0) ccw
  arc A25 (-3.2424, -4.0966) -> (-3.2887, -3.4262) centre (-3.635, -3.7869) ccw
  line L12 (-3.2424, -4.0966) -> (-3.4986, -4.4214)
  spline S12 degree 5 poles (-3.4986, -4.4214) (-3.5011, -4.4245) (-3.5059, -4.4309) (-3.5129, -4.4406) (-3.5216, -4.454) (-3.5317, -4.4713) (-3.5412, -4.4891) (-3.5504, -4.5071) (-3.5594, -4.5252) (-3.5682, -4.5434) (-3.5769, -4.5618) (-3.5854, -4.5803) (-3.5936, -4.599) (-3.6016, -4.6178) (-3.6093, -4.6369) (-3.6167, -4.6561) (-3.6239, -4.6755) (-3.6308, -4.695) (-3.6376, -4.7146) (-3.6442, -4.7344) (-3.6507, -4.7542) (-3.657, -4.7742) (-3.6631, -4.7943) (-3.669, -4.8144) (-3.6747, -4.8348) (-3.6802, -4.8552) (-3.6856, -4.8757) (-3.6907, -4.8963) (-3.6957, -4.917) (-3.7006, -4.9378) (-3.7053, -4.9587) (-3.7098, -4.9797) (-3.7142, -5.0008) (-3.7184, -5.022) (-3.7224, -5.0432) (-3.7263, -5.0646) (-3.73, -5.086) (-3.7335, -5.1075) (-3.7369, -5.1291) (-3.7402, -5.1508) (-3.7433, -5.1725) (-3.7462, -5.1943) (-3.749, -5.2162) (-3.7517, -5.2381) (-3.7542, -5.2602) (-3.7565, -5.2823) (-3.7587, -5.3044) (-3.7608, -5.3267) (-3.7627, -5.349) (-3.7644, -5.3713) (-3.766, -5.3937) (-3.7675, -5.4162) (-3.7688, -5.4388) (-3.77, -5.4614) (-3.771, -5.4841) (-3.7719, -5.5068) (-3.7726, -5.5296) (-3.7732, -5.5524) (-3.7737, -5.5753) (-3.774, -5.5982) (-3.7742, -5.6212) (-3.7742, -5.6443) (-3.7741, -5.6674) (-3.7739, -5.6906) (-3.7735, -5.7138) (-3.773, -5.737) (-3.7723, -5.7603) (-3.7715, -5.7836) (-3.7705, -5.807) (-3.7694, -5.8305) (-3.7682, -5.8539) (-3.7671, -5.8728) (-3.7663, -5.8869) (-3.7656, -5.8963) (-3.7653, -5.901) knots 0 0 0 0 0 0 0.01428571 0.02857143 0.04285714 0.05714286 0.07142857 0.08571429 0.1 0.11428571 0.12857143 0.14285714 0.15714286 0.17142857 0.18571429 0.2 0.21428571 0.22857143 0.24285714 0.25714286 0.27142857 0.28571429 0.3 0.31428571 0.32857143 0.34285714 0.35714286 0.37142857 0.38571429 0.4 0.41428571 0.42857143 0.44285714 0.45714286 0.47142857 0.48571429 0.5 0.51428571 0.52857143 0.54285714 0.55714286 0.57142857 0.58571429 0.6 0.61428571 0.62857143 0.64285714 0.65714286 0.67142857 0.68571429 0.7 0.71428571 0.72857143 0.74285714 0.75714286 0.77142857 0.78571429 0.8 0.81428571 0.82857143 0.84285714 0.85714286 0.87142857 0.88571429 0.9 0.91428571 0.92857143 0.94285714 0.95714286 0.97142857 0.98571429 1 1 1 1 1 1
  arc A26 (-3.7653, -5.901) -> (-3.2278, -6.2114) centre (0, 0) ccw
  spline S13 degree 5 poles (-2.0798, -5.2406) (-2.0812, -5.2443) (-2.0843, -5.2517) (-2.0893, -5.2626) (-2.0965, -5.2768) (-2.1064, -5.2942) (-2.117, -5.3113) (-2.128, -5.3283) (-2.1393, -5.3451) (-2.1506, -5.3619) (-2.1622, -5.3786) (-2.174, -5.3952) (-2.186, -5.4117) (-2.1983, -5.428) (-2.211, -5.4442) (-2.2239, -5.4602) (-2.2372, -5.4761) (-2.2506, -5.4919) (-2.2642, -5.5076) (-2.278, -5.5232) (-2.2919, -5.5387) (-2.3061, -5.5541) (-2.3204, -5.5694) (-2.3349, -5.5846) (-2.3497, -5.5997) (-2.3646, -5.6147) (-2.3797, -5.6296) (-2.395, -5.6444) (-2.4104, -5.6591) (-2.426, -5.6737) (-2.4418, -5.6882) (-2.4577, -5.7026) (-2.4738, -5.717) (-2.49, -5.7312) (-2.5064, -5.7453) (-2.5229, -5.7593) (-2.5396, -5.7733) (-2.5565, -5.7871) (-2.5735, -5.8008) (-2.5906, -5.8145) (-2.6079, -5.828) (-2.6253, -5.8415) (-2.6428, -5.8549) (-2.6605, -5.8681) (-2.6784, -5.8813) (-2.6963, -5.8944) (-2.7144, -5.9074) (-2.7326, -5.9203) (-2.751, -5.9331) (-2.7695, -5.9458) (-2.7881, -5.9584) (-2.8068, -5.9709) (-2.8257, -5.9833) (-2.8447, -5.9956) (-2.8638, -6.0078) (-2.8831, -6.02) (-2.9024, -6.032) (-2.9219, -6.0439) (-2.9415, -6.0558) (-2.9612, -6.0675) (-2.981, -6.0792) (-3.001, -6.0907) (-3.0211, -6.1022) (-3.0412, -6.1135) (-3.0615, -6.1248) (-3.0819, -6.136) (-3.1024, -6.147) (-3.123, -6.158) (-3.1438, -6.1689) (-3.1646, -6.1797) (-3.1856, -6.1903) (-3.2024, -6.1988) (-3.2151, -6.2051) (-3.2235, -6.2093) (-3.2278, -6.2114) knots 0 0 0 0 0 0 0.01428571 0.02857143 0.04285714 0.05714286 0.07142857 0.08571429 0.1 0.11428571 0.12857143 0.14285714 0.15714286 0.17142857 0.18571429 0.2 0.21428571 0.22857143 0.24285714 0.25714286 0.27142857 0.28571429 0.3 0.31428571 0.32857143 0.34285714 0.35714286 0.37142857 0.38571429 0.4 0.41428571 0.42857143 0.44285714 0.45714286 0.47142857 0.48571429 0.5 0.51428571 0.52857143 0.54285714 0.55714286 0.57142857 0.58571429 0.6 0.61428571 0.62857143 0.64285714 0.65714286 0.67142857 0.68571429 0.7 0.71428571 0.72857143 0.74285714 0.75714286 0.77142857 0.78571429 0.8 0.81428571 0.82857143 0.84285714 0.85714286 0.87142857 0.88571429 0.9 0.91428571 0.92857143 0.94285714 0.95714286 0.97142857 0.98571429 1 1 1 1 1 1
  line L13 (-2.0798, -5.2406) -> (-1.9265, -4.8563)
  arc A27 (-1.3228, -4.5613) -> (-1.9265, -4.8563) centre (-1.4621, -5.0415) ccw
  arc A28 (-1.3228, -4.5613) -> (-1.135, -4.6116) centre (0, 0) ccw
  arc A29 (-0.7597, -5.1689) -> (-1.135, -4.6116) centre (-1.2545, -5.0971) ccw
  line L14 (-0.7597, -5.1689) -> (-0.8192, -5.5783)
  spline S14 degree 5 poles (-0.8192, -5.5783) (-0.8197, -5.5823) (-0.8208, -5.5902) (-0.8219, -5.6021) (-0.8228, -5.6181) (-0.8229, -5.6381) (-0.8223, -5.6583) (-0.8212, -5.6784) (-0.8199, -5.6986) (-0.8184, -5.7188) (-0.8168, -5.7391) (-0.8149, -5.7593) (-0.8127, -5.7796) (-0.8102, -5.7999) (-0.8073, -5.8203) (-0.8041, -5.8406) (-0.8006, -5.861) (-0.7969, -5.8814) (-0.793, -5.9018) (-0.7888, -5.9222) (-0.7845, -5.9426) (-0.7799, -5.9631) (-0.7752, -5.9835) (-0.7702, -6.0039) (-0.765, -6.0244) (-0.7596, -6.0448) (-0.7539, -6.0653) (-0.7481, -6.0857) (-0.7421, -6.1061) (-0.7359, -6.1266) (-0.7295, -6.147) (-0.7229, -6.1675) (-0.7161, -6.1879) (-0.7092, -6.2083) (-0.7021, -6.2288) (-0.6947, -6.2492) (-0.6873, -6.2696) (-0.6796, -6.29) (-0.6717, -6.3104) (-0.6637, -6.3308) (-0.6555, -6.3512) (-0.6472, -6.3715) (-0.6387, -6.3919) (-0.63, -6.4122) (-0.6211, -6.4325) (-0.6121, -6.4528) (-0.6029, -6.4731) (-0.5936, -6.4934) (-0.5841, -6.5137) (-0.5744, -6.5339) (-0.5646, -6.5541) (-0.5546, -6.5743) (-0.5445, -6.5945) (-0.5342, -6.6147) (-0.5238, -6.6348) (-0.5132, -6.655) (-0.5024, -6.6751) (-0.4915, -6.6951) (-0.4805, -6.7152) (-0.4693, -6.7352) (-0.4579, -6.7552) (-0.4464, -6.7752) (-0.4348, -6.7952) (-0.423, -6.8151) (-0.4111, -6.835) (-0.399, -6.8549) (-0.3867, -6.8747) (-0.3744, -6.8945) (-0.3619, -6.9143) (-0.3492, -6.9341) (-0.3364, -6.9538) (-0.3261, -6.9695) (-0.3182, -6.9813) (-0.313, -6.9892) (-0.3103, -6.9931) knots 0 0 0 0 0 0 0.01428571 0.02857143 0.04285714 0.05714286 0.07142857 0.08571429 0.1 0.11428571 0.12857143 0.14285714 0.15714286 0.17142857 0.18571429 0.2 0.21428571 0.22857143 0.24285714 0.25714286 0.27142857 0.28571429 0.3 0.31428571 0.32857143 0.34285714 0.35714286 0.37142857 0.38571429 0.4 0.41428571 0.42857143 0.44285714 0.45714286 0.47142857 0.48571429 0.5 0.51428571 0.52857143 0.54285714 0.55714286 0.57142857 0.58571429 0.6 0.61428571 0.62857143 0.64285714 0.65714286 0.67142857 0.68571429 0.7 0.71428571 0.72857143 0.74285714 0.75714286 0.77142857 0.78571429 0.8 0.81428571 0.82857143 0.84285714 0.85714286 0.87142857 0.88571429 0.9 0.91428571 0.92857143 0.94285714 0.95714286 0.97142857 0.98571429 1 1 1 1 1 1
  arc A30 (-0.3103, -6.9931) -> (0.3103, -6.9931) centre (0, 0) ccw
  spline S15 degree 5 poles (0.8192, -5.5783) (0.8197, -5.5823) (0.8208, -5.5902) (0.8219, -5.6021) (0.8228, -5.6181) (0.8229, -5.6381) (0.8223, -5.6583) (0.8212, -5.6784) (0.8199, -5.6986) (0.8184, -5.7188) (0.8168, -5.7391) (0.8149, -5.7593) (0.8127, -5.7796) (0.8102, -5.7999) (0.8073, -5.8203) (0.8041, -5.8406) (0.8006, -5.861) (0.7969, -5.8814) (0.793, -5.9018) (0.7888, -5.9222) (0.7845, -5.9426) (0.7799, -5.9631) (0.7752, -5.9835) (0.7702, -6.0039) (0.765, -6.0244) (0.7596, -6.0448) (0.7539, -6.0653) (0.7481, -6.0857) (0.7421, -6.1061) (0.7359, -6.1266) (0.7295, -6.147) (0.7229, -6.1675) (0.7161, -6.1879) (0.7092, -6.2083) (0.7021, -6.2288) (0.6947, -6.2492) (0.6873, -6.2696) (0.6796, -6.29) (0.6717, -6.3104) (0.6637, -6.3308) (0.6555, -6.3512) (0.6472, -6.3715) (0.6387, -6.3919) (0.63, -6.4122) (0.6211, -6.4325) (0.6121, -6.4528) (0.6029, -6.4731) (0.5936, -6.4934) (0.5841, -6.5137) (0.5744, -6.5339) (0.5646, -6.5541) (0.5546, -6.5743) (0.5445, -6.5945) (0.5342, -6.6147) (0.5238, -6.6348) (0.5132, -6.655) (0.5024, -6.6751) (0.4915, -6.6951) (0.4805, -6.7152) (0.4693, -6.7352) (0.4579, -6.7552) (0.4464, -6.7752) (0.4348, -6.7952) (0.423, -6.8151) (0.4111, -6.835) (0.399, -6.8549) (0.3867, -6.8747) (0.3744, -6.8945) (0.3619, -6.9143) (0.3492, -6.9341) (0.3364, -6.9538) (0.3261, -6.9695) (0.3182, -6.9813) (0.313, -6.9892) (0.3103, -6.9931) knots 0 0 0 0 0 0 0.01428571 0.02857143 0.04285714 0.05714286 0.07142857 0.08571429 0.1 0.11428571 0.12857143 0.14285714 0.15714286 0.17142857 0.18571429 0.2 0.21428571 0.22857143 0.24285714 0.25714286 0.27142857 0.28571429 0.3 0.31428571 0.32857143 0.34285714 0.35714286 0.37142857 0.38571429 0.4 0.41428571 0.42857143 0.44285714 0.45714286 0.47142857 0.48571429 0.5 0.51428571 0.52857143 0.54285714 0.55714286 0.57142857 0.58571429 0.6 0.61428571 0.62857143 0.64285714 0.65714286 0.67142857 0.68571429 0.7 0.71428571 0.72857143 0.74285714 0.75714286 0.77142857 0.78571429 0.8 0.81428571 0.82857143 0.84285714 0.85714286 0.87142857 0.88571429 0.9 0.91428571 0.92857143 0.94285714 0.95714286 0.97142857 0.98571429 1 1 1 1 1 1
  line L15 (0.8192, -5.5783) -> (0.7597, -5.1689)
  arc A31 (1.135, -4.6116) -> (0.7597, -5.1689) centre (1.2545, -5.0971) ccw
  arc A32 (1.135, -4.6116) -> (1.3228, -4.5613) centre (0, 0) ccw
  arc A33 (1.9265, -4.8563) -> (1.3228, -4.5613) centre (1.4621, -5.0415) ccw
  line L16 (1.9265, -4.8563) -> (2.0798, -5.2406)
  spline S16 degree 5 poles (2.0798, -5.2406) (2.0812, -5.2443) (2.0843, -5.2517) (2.0893, -5.2626) (2.0965, -5.2768) (2.1064, -5.2942) (2.117, -5.3113) (2.128, -5.3283) (2.1393, -5.3451) (2.1506, -5.3619) (2.1622, -5.3786) (2.174, -5.3952) (2.186, -5.4117) (2.1983, -5.428) (2.211, -5.4442) (2.2239, -5.4602) (2.2372, -5.4761) (2.2506, -5.4919) (2.2642, -5.5076) (2.278, -5.5232) (2.2919, -5.5387) (2.3061, -5.5541) (2.3204, -5.5694) (2.3349, -5.5846) (2.3497, -5.5997) (2.3646, -5.6147) (2.3797, -5.6296) (2.395, -5.6444) (2.4104, -5.6591) (2.426, -5.6737) (2.4418, -5.6882) (2.4577, -5.7026) (2.4738, -5.717) (2.49, -5.7312) (2.5064, -5.7453) (2.5229, -5.7593) (2.5396, -5.7733) (2.5565, -5.7871) (2.5735, -5.8008) (2.5906, -5.8145) (2.6079, -5.828) (2.6253, -5.8415) (2.6428, -5.8549) (2.6605, -5.8681) (2.6784, -5.8813) (2.6963, -5.8944) (2.7144, -5.9074) (2.7326, -5.9203) (2.751, -5.9331) (2.7695, -5.9458) (2.7881, -5.9584) (2.8068, -5.9709) (2.8257, -5.9833) (2.8447, -5.9956) (2.8638, -6.0078) (2.8831, -6.02) (2.9024, -6.032) (2.9219, -6.0439) (2.9415, -6.0558) (2.9612, -6.0675) (2.981, -6.0792) (3.001, -6.0907) (3.0211, -6.1022) (3.0412, -6.1135) (3.0615, -6.1248) (3.0819, -6.136) (3.1024, -6.147) (3.123, -6.158) (3.1438, -6.1689) (3.1646, -6.1797) (3.1856, -6.1903) (3.2024, -6.1988) (3.2151, -6.2051) (3.2235, -6.2093) (3.2278, -6.2114) knots 0 0 0 0 0 0 0.01428571 0.02857143 0.04285714 0.05714286 0.07142857 0.08571429 0.1 0.11428571 0.12857143 0.14285714 0.15714286 0.17142857 0.18571429 0.2 0.21428571 0.22857143 0.24285714 0.25714286 0.27142857 0.28571429 0.3 0.31428571 0.32857143 0.34285714 0.35714286 0.37142857 0.38571429 0.4 0.41428571 0.42857143 0.44285714 0.45714286 0.47142857 0.48571429 0.5 0.51428571 0.52857143 0.54285714 0.55714286 0.57142857 0.58571429 0.6 0.61428571 0.62857143 0.64285714 0.65714286 0.67142857 0.68571429 0.7 0.71428571 0.72857143 0.74285714 0.75714286 0.77142857 0.78571429 0.8 0.81428571 0.82857143 0.84285714 0.85714286 0.87142857 0.88571429 0.9 0.91428571 0.92857143 0.94285714 0.95714286 0.97142857 0.98571429 1 1 1 1 1 1
  arc A34 (3.2278, -6.2114) -> (3.7653, -5.901) centre (0, 0) ccw
  spline S17 degree 5 poles (3.4986, -4.4214) (3.5011, -4.4245) (3.5059, -4.4309) (3.5129, -4.4406) (3.5216, -4.454) (3.5317, -4.4713) (3.5412, -4.4891) (3.5504, -4.5071) (3.5594, -4.5252) (3.5682, -4.5434) (3.5769, -4.5618) (3.5854, -4.5803) (3.5936, -4.599) (3.6016, -4.6178) (3.6093, -4.6369) (3.6167, -4.6561) (3.6239, -4.6755) (3.6308, -4.695) (3.6376, -4.7146) (3.6442, -4.7344) (3.6507, -4.7542) (3.657, -4.7742) (3.6631, -4.7943) (3.669, -4.8144) (3.6747, -4.8348) (3.6802, -4.8552) (3.6856, -4.8757) (3.6907, -4.8963) (3.6957, -4.917) (3.7006, -4.9378) (3.7053, -4.9587) (3.7098, -4.9797) (3.7142, -5.0008) (3.7184, -5.022) (3.7224, -5.0432) (3.7263, -5.0646) (3.73, -5.086) (3.7335, -5.1075) (3.7369, -5.1291) (3.7402, -5.1508) (3.7433, -5.1725) (3.7462, -5.1943) (3.749, -5.2162) (3.7517, -5.2381) (3.7542, -5.2602) (3.7565, -5.2823) (3.7587, -5.3044) (3.7608, -5.3267) (3.7627, -5.349) (3.7644, -5.3713) (3.766, -5.3937) (3.7675, -5.4162) (3.7688, -5.4388) (3.77, -5.4614) (3.771, -5.4841) (3.7719, -5.5068) (3.7726, -5.5296) (3.7732, -5.5524) (3.7737, -5.5753) (3.774, -5.5982) (3.7742, -5.6212) (3.7742, -5.6443) (3.7741, -5.6674) (3.7739, -5.6906) (3.7735, -5.7138) (3.773, -5.737) (3.7723, -5.7603) (3.7715, -5.7836) (3.7705, -5.807) (3.7694, -5.8305) (3.7682, -5.8539) (3.7671, -5.8728) (3.7663, -5.8869) (3.7656, -5.8963) (3.7653, -5.901) knots 0 0 0 0 0 0 0.01428571 0.02857143 0.04285714 0.05714286 0.07142857 0.08571429 0.1 0.11428571 0.12857143 0.14285714 0.15714286 0.17142857 0.18571429 0.2 0.21428571 0.22857143 0.24285714 0.25714286 0.27142857 0.28571429 0.3 0.31428571 0.32857143 0.34285714 0.35714286 0.37142857 0.38571429 0.4 0.41428571 0.42857143 0.44285714 0.45714286 0.47142857 0.48571429 0.5 0.51428571 0.52857143 0.54285714 0.55714286 0.57142857 0.58571429 0.6 0.61428571 0.62857143 0.64285714 0.65714286 0.67142857 0.68571429 0.7 0.71428571 0.72857143 0.74285714 0.75714286 0.77142857 0.78571429 0.8 0.81428571 0.82857143 0.84285714 0.85714286 0.87142857 0.88571429 0.9 0.91428571 0.92857143 0.94285714 0.95714286 0.97142857 0.98571429 1 1 1 1 1 1
  line L17 (3.4986, -4.4214) -> (3.2424, -4.0966)
  arc A35 (3.2887, -3.4262) -> (3.2424, -4.0966) centre (3.635, -3.7869) ccw
  arc A36 (3.2887, -3.4262) -> (3.4262, -3.2887) centre (0, 0) ccw
  arc A37 (4.0966, -3.2424) -> (3.4262, -3.2887) centre (3.7869, -3.635) ccw
  line L18 (4.0966, -3.2424) -> (4.4214, -3.4986)
  spline S18 degree 5 poles (4.4214, -3.4986) (4.4245, -3.5011) (4.4309, -3.5059) (4.4406, -3.5129) (4.454, -3.5216) (4.4713, -3.5317) (4.4891, -3.5412) (4.5071, -3.5504) (4.5252, -3.5594) (4.5434, -3.5682) (4.5618, -3.5769) (4.5803, -3.5854) (4.599, -3.5936) (4.6178, -3.6016) (4.6369, -3.6093) (4.6561, -3.6167) (4.6755, -3.6239) (4.695, -3.6308) (4.7146, -3.6376) (4.7344, -3.6442) (4.7542, -3.6507) (4.7742, -3.657) (4.7943, -3.6631) (4.8144, -3.669) (4.8348, -3.6747) (4.8552, -3.6802) (4.8757, -3.6856) (4.8963, -3.6907) (4.917, -3.6957) (4.9378, -3.7006) (4.9587, -3.7053) (4.9797, -3.7098) (5.0008, -3.7142) (5.022, -3.7184) (5.0432, -3.7224) (5.0646, -3.7263) (5.086, -3.73) (5.1075, -3.7335) (5.1291, -3.7369) (5.1508, -3.7402) (5.1725, -3.7433) (5.1943, -3.7462) (5.2162, -3.749) (5.2381, -3.7517) (5.2602, -3.7542) (5.2823, -3.7565) (5.3044, -3.7587) (5.3267, -3.7608) (5.349, -3.7627) (5.3713, -3.7644) (5.3937, -3.766) (5.4162, -3.7675) (5.4388, -3.7688) (5.4614, -3.77) (5.4841, -3.771) (5.5068, -3.7719) (5.5296, -3.7726) (5.5524, -3.7732) (5.5753, -3.7737) (5.5982, -3.774) (5.6212, -3.7742) (5.6443, -3.7742) (5.6674, -3.7741) (5.6906, -3.7739) (5.7138, -3.7735) (5.737, -3.773) (5.7603, -3.7723) (5.7836, -3.7715) (5.807, -3.7705) (5.8305, -3.7694) (5.8539, -3.7682) (5.8728, -3.7671) (5.8869, -3.7663) (5.8963, -3.7656) (5.901, -3.7653) knots 0 0 0 0 0 0 0.01428571 0.02857143 0.04285714 0.05714286 0.07142857 0.08571429 0.1 0.11428571 0.12857143 0.14285714 0.15714286 0.17142857 0.18571429 0.2 0.21428571 0.22857143 0.24285714 0.25714286 0.27142857 0.28571429 0.3 0.31428571 0.32857143 0.34285714 0.35714286 0.37142857 0.38571429 0.4 0.41428571 0.42857143 0.44285714 0.45714286 0.47142857 0.48571429 0.5 0.51428571 0.52857143 0.54285714 0.55714286 0.57142857 0.58571429 0.6 0.61428571 0.62857143 0.64285714 0.65714286 0.67142857 0.68571429 0.7 0.71428571 0.72857143 0.74285714 0.75714286 0.77142857 0.78571429 0.8 0.81428571 0.82857143 0.84285714 0.85714286 0.87142857 0.88571429 0.9 0.91428571 0.92857143 0.94285714 0.95714286 0.97142857 0.98571429 1 1 1 1 1 1